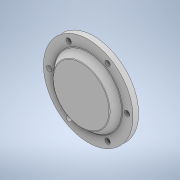
# Autodesk Inventor part: 轴承端盖2
Saved by Autodesk Inventor 2020 (Build 240168000, 168)
## iProperties
Created: 2021-06-16
Part Number: 轴承端盖2
Material: 常规
Document SubType Name: Modeling
Designer: dell
Density: 1 g/cm^3
Appearance: 默认
Author: dell
Autodesk Inventor part; units mm, degrees
ref_plane "YZ Plane" through (0, 0, 0) normal (1, 0, 0) x (0, 1, 0)
ref_plane "XZ Plane" through (0, 0, 0) normal (0, 1, 0) x (-1, 0, 0)
ref_plane "XY Plane" through (0, 0, 0) normal (0, 0, 1) x (1, 0, 0)
ref_plane "工作平面1" through (0, 0, 0) normal (0, 0, 1) x (1, 0, 0)
sketch "草图1" plane through (0, 0, 0) normal (0, 0, 1) x (1, 0, 0)
  arc A0 (-47.5, -70) -> (-47.5, 70) centre (-47.5, 0) ccw construction
  circle A1 centre (-47.5, 0) radius 82.5 construction
  arc A2 (-47.5, -95) -> (-47.5, 95) centre (-47.5, 0) ccw construction
  line L0 (-47.5, 70) -> (-47.5, 95) construction
  arc A3 (-47.5, -70) -> (-47.5, 70) centre (-47.5, 0) ccw construction
  line L1 (-47.5, -95) -> (-47.5, -70) construction
  arc A4 (-47.5, -70) -> (-47.5, 70) centre (-47.5, 0) ccw construction
  circle A5 centre (-47.5, 0) radius 95
  circle A6 centre (-130, 0) radius 5.5
  line L2 (-180.5, 0) -> (85.5, 0) construction
  circle A7 centre (-88.75, -71.4471) radius 5.5
  circle A8 centre (-6.25, -71.4471) radius 5.5
  circle A9 centre (35, 0) radius 5.5
  circle A10 centre (-6.25, 71.4471) radius 5.5
  circle A11 centre (-88.75, 71.4471) radius 5.5
  point P0 (0, 0)
  dimension "d0" = 165
  dimension "d1" = 11
  dimension "d4" = 360
  constraints: 7 centre point, 2 coincident, 1 concentric, 1 horizontal alignment, 1 point on line, 15 other
  measures "d1" diameter of A6
extrude "拉伸1" add sketch "草图1" along normal blind 12
sketch "草图2" plane through (-47.5, 0, 0) normal (0, 0, -1) x (-1, 0, 0)
  arc A0 (0, 70) -> (0, -70) centre (0, 0) ccw construction
  circle A1 centre (0, 0) radius 70
  circle A2 centre (0, 0) radius 60
  point P0 (-47.5, 0)
  dimension "d8" = 10
  constraints: 2 centre point, 1 coincident, 1 concentric
  measures "d8" radial gap between concentric circles of A1 A2
extrude "拉伸2" add sketch "草图2" along normal blind 10.5
sketch "草图3" plane through (-47.5, 0, 12) normal (0, 0, 1) x (1, 0, 0)
  circle A0 centre (0, 0) radius 70 construction
  circle A1 centre (0, 0) radius 70 construction
  circle A2 centre (0, 0) radius 72
  point P0 (47.5, 0)
  dimension "d11" = 2
  constraints: 1 centre point
  measures "d11" radial gap between concentric circles of A0 A2
ref_plane "工作平面2" through (-47.5, 0, 27) normal (0, 0, 1) x (1, 0, 0)
sketch "草图4" plane through (-47.5, 0, 27) normal (0, 0, 1) x (1, 0, 0)
  circle A0 centre (0, 0) radius 72 construction
  circle A1 centre (0, 0) radius 60 projected
  point P0 (47.5, 0)
loft "放样1" add profiles "草图3", "草图4"
sketch "草图5" plane through (-47.5, 0, 0) normal (0, 0, -1) x (-1, 0, 0)
  circle A0 centre (0, 0) radius 60 projected
  point P0 (-47.5, 0)
extrude "拉伸3" cut sketch "草图5" against normal blind 5
fillet "圆角1" radius 2 2 edges at (-107.5, 0, 27) (-119.5, 0, 12)
